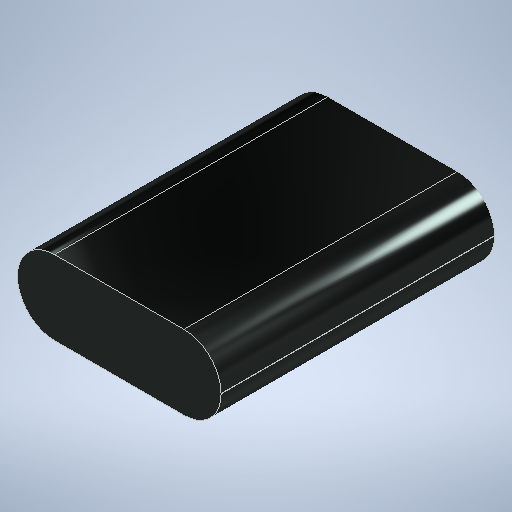
# Autodesk Inventor part: PI4_housing
Saved by Autodesk Inventor 2025 (Build 290162000, 162)
## iProperties
Created: 2024-09-26
Part Number: PI4_housing
Material: Generic
Document SubType Name: Modeling
Designer: DANIEL
Density: 1 g/cm^3
Appearance: Gunmetal - Polished
Author: DANIEL
Autodesk Inventor part; units mm, degrees
ref_plane "YZ Plane" through (0, 0, 0) normal (1, 0, 0) x (0, 1, 0)
ref_plane "XZ Plane" through (0, 0, 0) normal (0, 1, 0) x (-1, 0, 0)
ref_plane "XY Plane" through (0, 0, 0) normal (0, 0, 1) x (1, 0, 0)
sketch "Sketch1" plane through (0, 0, 0) normal (0, 1, 0) x (-1, 0, 0)
  line L0 (33.5, -45) -> (-33.5, -45)
  line L1 (-33.5, -45) -> (-33.5, 45)
  line L2 (-33.5, 45) -> (33.5, 45)
  line L3 (33.5, 45) -> (33.5, -45)
  line L4 (33.5, -45) -> (-33.5, 45) construction
  line L5 (-33.5, -45) -> (33.5, 45) construction
  point P0 (0, 0)
  dimension "d0" = 67
  dimension "d1" = 90
  constraints: 12 end point, 2 midpoint, 2 parallel, 1 horizontal, 1 perpendicular
  measures "d0" distance of L1.end L2.end
  measures "d1" distance of L0.end L1.end
extrude "Extrusion1" add sketch "Sketch1" along normal blind 24.5
fillet "Fillet2" radius 12.2 4 edges at (33.5, 24.5, 0) (33.5, 0, 0) (-33.5, 24.5, 0) (-33.5, 0, 0)
body "Solid1"
